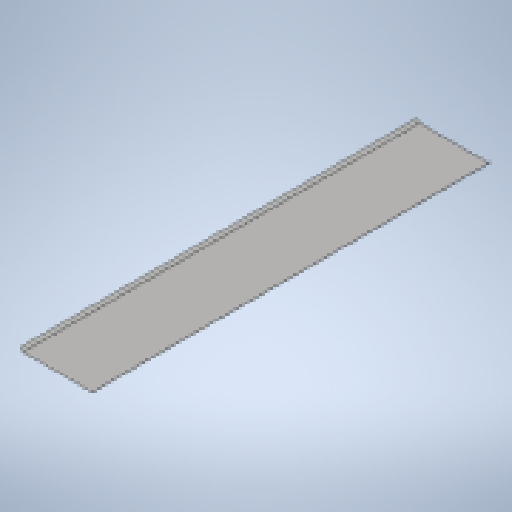
# Autodesk Inventor part: MSC 0107 sheet gills
Saved by Autodesk Inventor 2025 (Build 290162010, 162A)
## iProperties
Created: 2024-06-15
Part Number: MSC 0107 sheet gills
Material: Stainless Steel
Document SubType Name: Sheet Metal
Designer: pokla
Stock Number: МОО 0101 лист жабра
Mass: 8000 g
Surface Area: 40030 cm^2
Volume: 1000 cm^3
Density: 8 g/cm^3
Sheet Metal Rule: Default_mm
Appearance: Default
Author: pokla
Autodesk Inventor part; units mm, degrees
ref_plane "YZ Plane" through (0, 0, 0) normal (1, 0, 0) x (0, 1, 0)
ref_plane "XZ Plane" through (0, 0, 0) normal (0, 1, 0) x (-1, 0, 0)
ref_plane "XY Plane" through (0, 0, 0) normal (0, 0, 1) x (1, 0, 0)
sketch "Sketch6" plane through (0, 0, 0) normal (0, 1, 0) x (-1, 0, 0)
  line L0 (175, -1000) -> (-175, -1000)
  line L1 (-175, -1000) -> (-175, 1000)
  line L2 (-175, 1000) -> (175, 1000)
  line L3 (175, 1000) -> (175, -1000)
  line L4 (175, -1000) -> (-175, 1000) construction
  line L5 (-175, -1000) -> (175, 1000) construction
  point P0 (0, 0)
  dimension "d52" = 350
  dimension "d53" = 2000
  measures "d52" distance of L1.end L2.end
  measures "d53" distance of L0.end L1.end
extrude "Plate2" add sketch "Sketch6" along normal blind 0.5
sketch "Sketch10" plane through (-174.6343, 0.341, 1000) normal (-0.7313537, -0.6819984, 0) x (0.6819984, -0.7313537, 0)
  line L0 (0, -2000) -> (0, 0)
  line L1 (0, 0) -> (-20, 0)
  line L2 (-20, 0) -> (-20, -2000)
  line L3 (-20, -2000) -> (0, -2000)
  constraints: 6 end point, 1 horizontal, 1 perpendicular, 1 vertical
edge flange "Flange1" height 20 angle 47 thickness 0.5 bend radius 0.5 thickness toward (-0.7313537, -0.6819984, 0) relief straight relief width 0.5 relief depth 0.25 edges at (-175, 0.5, 0) wall of the first edge with corners at (-174.6343, 0.341, -1000) (-174.6343, 0.341, 1000) (-188.2743, 14.9681, 1000) (-188.2743, 14.9681, -1000)
bend "Bend2"
corner "Corner2"
sketch "Sketch11" plane through (174.659, 0.3657, -1000) normal (0.6819984, -0.7313537, 0) x (0.7313537, 0.6819984, 0)
  line L0 (0, 2000) -> (0, 0)
  line L1 (0, 0) -> (20, 0)
  line L2 (20, 0) -> (20, 2000)
  line L3 (20, 2000) -> (0, 2000)
  constraints: 6 end point, 1 horizontal, 1 perpendicular, 1 vertical
edge flange "Flange2" height 20 angle 43 thickness 0.5 bend radius 0.5 thickness toward (0.6819984, -0.7313537, 0) relief straight relief width 0.5 relief depth 0.25 edges at (175, 0.5, 0) wall of the first edge with corners at (174.659, 0.3657, 1000) (174.659, 0.3657, -1000) (189.2861, 14.0056, -1000) (189.2861, 14.0056, 1000)
bend "Bend3"
corner "Corner3"
equation "\"d52\" = ЖАБРЫ_базовая_ширина - 5 * ЖАБРЫ_шаг"
equation "\"d53\" = ЖАБРЫ_базовая_длина_дл_лист"
equation "\"d54\" = Thickness"
equation "\"d74\" = BendReliefWidth"
equation "\"d75\" = BendReliefDepth"
equation "\"d76\" = MinimumRemnant"
equation "\"d77\" = TransitionRadius"
equation "\"d80\" = BendRadius"
equation "\"d81\" = CornerReliefSize"
equation "\"d82\" = GapSize"
equation "\"d83\" = JacobiRadiusSize"
equation "\"d84\" = BendReliefWidth"
equation "\"d85\" = BendReliefDepth"
equation "\"d86\" = MinimumRemnant"
equation "\"d87\" = TransitionRadius"
equation "\"d90\" = BendRadius"
equation "\"d91\" = CornerReliefSize"
equation "\"d92\" = GapSize"
equation "\"d93\" = JacobiRadiusSize"
equation "\"BendRadius\" = Thickness"
equation "\"BendReliefWidth\" = Thickness"
equation "\"BendReliefDepth\" = 0.5 * Thickness"
equation "\"CornerReliefSize\" = 4 * Thickness"
equation "\"MinimumRemnant\" = 2 * Thickness"
equation "\"TransitionRadius\" = BendRadius"
equation "\"JacobiRadiusSize\" = BendRadius"
equation "\"GapSize\" = Thickness"
equation "\"ЖАБРЫ_базовая_ширина\" = 900"
equation "\"ЖАБРЫ_шаг\" = 110"
equation "\"ЖАБРЫ_базовая_длина_дл_лист\" = 2000"
equation "\"Thickness\" = 0.5"
body "Solid2"
